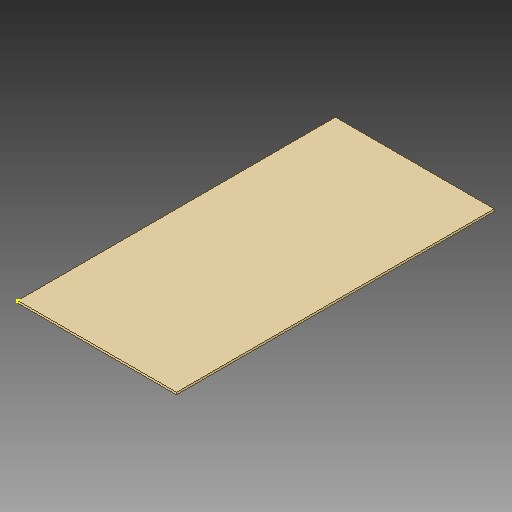
# Autodesk Inventor part: Lathhouse roof
Saved by Autodesk Inventor 2018 (Build 220112000, 112)
## iProperties
Created: 2019-05-09
Part Number: Lathhouse roof
Material: Generic
Document SubType Name: Sheet Metal
Designer: 10043883
Density: 1 g/cm^3
Appearance: Wheat
Sheet Metal Rule: Default_mm
Mass: 1.69901e+08 g
Surface Area: 1.36567e+07 cm^2
Volume: 1.69901e+08 cm^3
Author: 10043883
Autodesk Inventor part; units mm, degrees
ref_plane "YZ Plane" through (0, 0, 0) normal (1, 0, 0) x (0, 1, 0)
ref_plane "XZ Plane" through (0, 0, 0) normal (0, 1, 0) x (-1, 0, 0)
ref_plane "XY Plane" through (0, 0, 0) normal (0, 0, 1) x (1, 0, 0)
sketch "Sketch1" plane through (0, 0, 0) normal (0, 1, 0) x (-1, 0, 0)
  line L0 (0, 0) -> (-18288, 0)
  line L1 (-18288, 0) -> (-18288, -36576)
  line L2 (-18288, -36576) -> (0, -36576)
  line L3 (0, -36576) -> (0, 0)
  dimension "d0" = 18288
  dimension "d1" = 36576
  constraints: 8 end point, 2 parallel, 1 horizontal, 1 perpendicular
  measures "d0" distance of L2.end L1.end
  measures "d1" distance of L1.end L0.end
extrude "Extrusion1" add sketch "Sketch1" along normal blind 254
sketch "Sketch2" plane through (0, 254, 0) normal (0, 1, 0) x (1, 0, 0)
  point P0 (0, 0)
equation "\"BendRadius\" = Thickness"
equation "\"BendReliefWidth\" = Thickness"
equation "\"BendReliefDepth\" = 0.5 * Thickness"
equation "\"CornerReliefSize\" = 4 * Thickness"
equation "\"MinimumRemnant\" = 2 * Thickness"
equation "\"TransitionRadius\" = BendRadius"
equation "\"JacobiRadiusSize\" = BendRadius"
equation "\"GapSize\" = Thickness"
equation "\"Thickness\" = 0.5"
body "Solid1"
